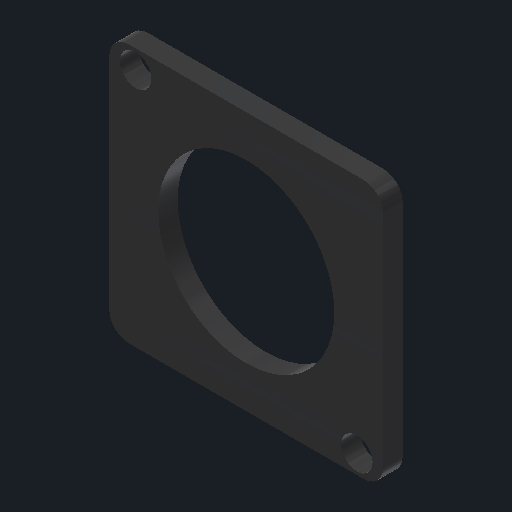
# Autodesk Inventor part: SPACER,NEO550,ARM
Saved by Autodesk Inventor 2025.1 (Build 291241020, 241B)
## iProperties
Category: _
Manager: _
ILogicPurgeVersion: 0.0.0.0
OnSaveVersion: 3.5.0.0
OnSaveAssembly: COREAutomationManager
Created: 2025-03-17
Part Number: SPACER,NEO550,ARM
Checked By: 00
Engr Approved By: _
User Status: Work In Process
Material: Nylon 6/6
Description: STANDARD (mm)
Document SubType Name: Modeling
Mfg Approved By: John.Thibert
Designer: John.Thibert
Manufacturer: Standard
Standards Organization: Custom
Mass: 4.22105 g
Surface Area: 32.7163 cm^2
Volume: 3.73544 cm^3
Density: 1.13 g/cm^3
Appearance: Dark Gray
CN_MASS: 0.0
CN_SERVICEABLE: _
FIRST_DESCRIPTION: _
SECOND_DESCRIPTION: _
THIRD_DESCRIPTION: _
ModelCat: Uncategorized
MaterialName: Nylon 6/6
Subject: _
Author: John.Thibert
Keywords: -
Revision Number: A
Autodesk Inventor part; units mm, degrees
ref_plane "YZ Plane" through (0, 0, 0) normal (1, 0, 0) x (0, 1, 0)
ref_plane "XZ Plane" through (0, 0, 0) normal (0, 1, 0) x (-1, 0, 0)
ref_plane "XY Plane" through (0, 0, 0) normal (0, 0, 1) x (1, 0, 0)
sketch "Sketch2" plane through (0, 0, 0) normal (0, 0, 1) x (1, 0, 0)
  line L0 (22.225, 21.0058) -> (-22.225, 21.0058)
  line L1 (-22.225, 21.0058) -> (-22.225, -21.0058)
  line L2 (-22.225, -21.0058) -> (22.225, -21.0058)
  line L3 (22.225, -21.0058) -> (22.225, 21.0058)
  line L4 (22.225, 21.0058) -> (-22.225, -21.0058) construction
  line L5 (-22.225, 21.0058) -> (22.225, -21.0058) construction
  point P0 (0, 0)
  dimension "d0" = 44.45
  dimension "d1" = 42.0116
  constraints: 12 end point, 2 midpoint, 2 parallel, 1 horizontal, 1 perpendicular
  measures "d0" distance of L2.end L1.end
  measures "d1" distance of L1.end L0.end
extrude "Extrusion1" add sketch "Sketch2" along normal mid plane 3.175
sketch "Sketch3" plane through (0, 0, 1.5875) normal (0, 0, 1) x (1, 0, 0)
  point P0 (0, 0)
  point P1 (0, 0)
  constraints: 1 coincident
hole "Hole1" at (0, 0, 1.5875) direction (0, 0, -1) diameter 28.575 end through all start extended yes
sketch "Sketch4" plane through (0, 0, 1.5875) normal (0, 0, 1) x (1, 0, 0)
  line L0 (17.9605, -17.9605) -> (-17.9605, 17.9605) construction
  line L1 (-31.115, 0) -> (31.115, 0) construction
  line L2 (0, 29.4081) -> (0, -29.4081) construction
  point P0 (0, 0)
  point P1 (0, 0)
  dimension "d1" = 42.0116
  dimension "d11" = 45
  dimension "d12" = 50.8
  constraints: 2 end point, 1 coincident, 1 midpoint
  measures "d11" angle of L2 L0
  measures "d12" distance of L0.start L0.end
hole "Hole2" at (17.9605, -17.9605, 1.5875) at (-17.9605, 17.9605, 1.5875) direction (0, 0, -1) diameter 5.1054 end through all start extended yes clearance for "Flat Head Machine Screw (82)" size "#10" standard "Ansi Unified Screw Threads"
fillet "Fillet1" radius 3.175 4 edges at (22.225, -21.0058, 0) (-22.225, 21.0058, 0) (22.225, 21.0058, 0) (-22.225, -21.0058, 0)
body "Solid1"
